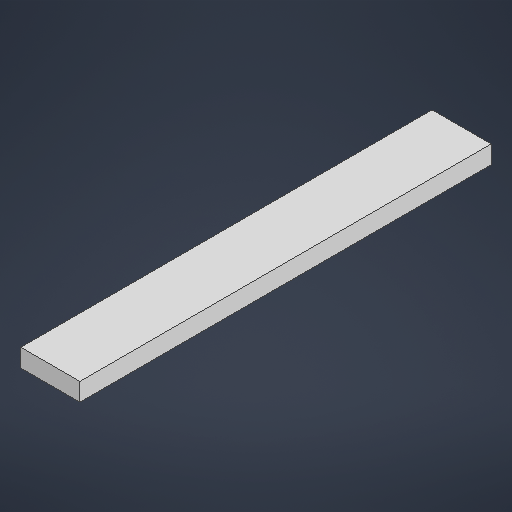
# Autodesk Inventor part: BasePlateipt
Saved by Autodesk Inventor 2026.2 (Build 302298000, 298)
## iProperties
Created: 2025-12-17
Part Number: BasePlateipt
Material: Generic
Document SubType Name: Modeling
Designer: Thoma
Density: 1 g/cm^3
Appearance: Default
Author: Thoma
Autodesk Inventor part; units mm, degrees
ref_plane "YZ Plane" through (0, 0, 0) normal (1, 0, 0) x (0, 1, 0)
ref_plane "XZ Plane" through (0, 0, 0) normal (0, 1, 0) x (-1, 0, 0)
ref_plane "XY Plane" through (0, 0, 0) normal (0, 0, 1) x (1, 0, 0)
sketch "Sketch1" plane through (0, 0, 0) normal (0, 1, 0) x (-1, 0, 0)
  line L0 (15.3846, 113.8462) -> (-7.6154, 113.8462)
  line L1 (-7.6154, 113.8462) -> (-7.6154, -46.1538)
  line L2 (-7.6154, -46.1538) -> (15.3846, -46.1538)
  line L3 (15.3846, -46.1538) -> (15.3846, 113.8462)
  point P0 (0, 0)
  dimension "d0" = 23
  dimension "d1" = 160
  constraints: 8 end point, 2 parallel, 1 horizontal, 1 perpendicular
  measures "d0" distance of L1.end L2.end
  measures "d1" distance of L2.end L0.start
extrude "Extrusion1" add sketch "Sketch1" along normal blind 7
body "Solid1"
